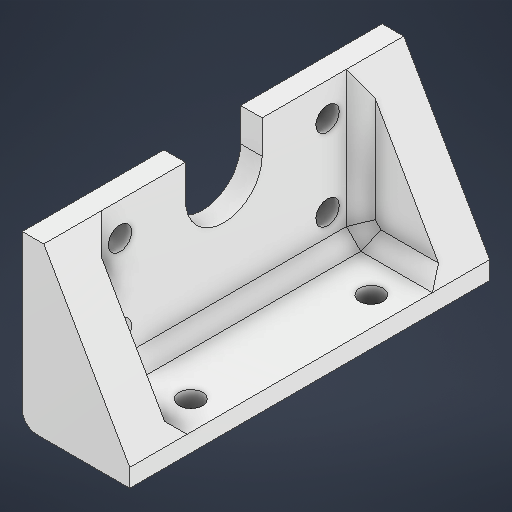
# Autodesk Inventor part: CNC-022-XAxisBallScrewStabilizerMount
Saved by Autodesk Inventor 2026.2 (Build 302298000, 298)
## iProperties
Created: 2026-06-24
Part Number: CNC-022-XAxisBallScrewStabilizerMount
Material: ABS Plastic
Document SubType Name: Modeling
Designer: Kenji
Density: 1.06 g/cm^3
Appearance: Smooth - White
Author: Kenji
Autodesk Inventor part; units mm, degrees
ref_plane "YZ Plane" through (0, 0, 0) normal (1, 0, 0) x (0, 1, 0)
ref_plane "XZ Plane" through (0, 0, 0) normal (0, 1, 0) x (-1, 0, 0)
ref_plane "XY Plane" through (0, 0, 0) normal (0, 0, 1) x (1, 0, 0)
sketch "Sketch1" plane through (0, 0, 0) normal (1, 0, 0) x (0, 1, 0)
  line L0 (-9, -23) -> (9, -23) construction
  line L1 (9, -23) -> (9, 23) construction
  line L2 (9, 23) -> (-9, 23) construction
  line L3 (-9, 23) -> (-9, -23) construction
  line L4 (-9, -23) -> (9, 23) construction
  line L5 (9, -23) -> (-9, 23) construction
  circle A0 centre (9, 23) radius 2.6
  circle A1 centre (9, -23) radius 2.6
  circle A2 centre (-9, -23) radius 2.6
  circle A3 centre (-9, 23) radius 2.6
  circle A4 centre (9, 23) radius 7.3625 construction
  circle A5 centre (9, -23) radius 7.3625 construction
  circle A6 centre (-9, -23) radius 7.3625 construction
  circle A7 centre (-9, 23) radius 7.3625 construction
  line L6 (16.3625, 30.3625) -> (-21, 30.3625)
  line L7 (-21, 30.3625) -> (-21, -30.3625)
  line L8 (-21, -30.3625) -> (16.3625, -30.3625)
  line L9 (16.3625, -30.3625) -> (16.3625, 30.3625)
  point P0 (0, 0)
  dimension "d0" = 5.2
  dimension "d1" = 46
  dimension "d2" = 18
  dimension "d3" = 4.7625
  dimension "d7" = 12
  constraints: 20 end point, 8 centre point, 7 coincident, 6 equal radius, 4 parallel, 3 tangent, 2 horizontal, 2 midpoint, 2 perpendicular
  measures "d0" diameter of A0
  measures "d1" distance of L0.end L1.end
  measures "d2" distance of L2.end L1.end
  measures "d3" radial gap between concentric circles of A4 A0
  measures "d7" distance from line of L7 L0.start
extrude "Extrusion1" add sketch "Sketch1" along normal blind 4.7625
sketch "Sketch4" plane through (4.7625, 0, 0) normal (1, 0, 0) x (0, 0, -1)
  arc A0 (-8.5, 9) -> (8.5, 9) centre (0, 9) ccw
  circle A1 centre (-23, 9) radius 2.6 projected
  line L0 (8.5, 9) -> (8.5, 16.3625)
  line L1 (30.3625, 16.3625) -> (-30.3625, 16.3625) projected
  line L2 (-8.5, 9) -> (-8.5, 16.3625)
  point P0 (0, 0)
  point P1 (27.1875, 16.3625)
  point P2 (-27.1875, 16.3625)
  dimension "d21" = 17
  constraints: 4 end point, 2 point on circle, 2 point on line, 2 tangent, 1 centre point, 1 horizontal alignment, 1 perpendicular, 1 vertical, 1 vertical alignment
  measures "d21" diameter of A0
extrude "Extrusion5" cut sketch "Sketch4" against normal through all contours L2 L1 L0 A0
sketch "Sketch5" plane through (4.7625, 0, 0) normal (1, 0, 0) x (0, 0, -1)
  line L0 (30.3625, 16.3625) -> (8.5, 16.3625) projected
  line L1 (-30.3625, 16.3625) -> (-30.3625, -21) projected
  line L2 (-30.3625, -21) -> (30.3625, -21) projected
  line L3 (30.3625, -21) -> (30.3625, 16.3625) projected
  line L4 (-8.5, 16.3625) -> (-30.3625, 16.3625) projected
  line L5 (8.5, 16.3625) -> (8.5, 9) projected
  arc A0 (-8.5, 9) -> (8.5, 9) centre (0, 9) ccw projected
  line L6 (-8.5, 9) -> (-8.5, 16.3625) projected
  circle A1 centre (-23, -9) radius 2.6 projected
  circle A2 centre (23, -9) radius 2.6 projected
  circle A3 centre (23, 9) radius 2.6 projected
  circle A4 centre (-23, 9) radius 2.6 projected
  line L7 (30.3625, -21) -> (30.3625, 13.1875) projected
  line L8 (-30.3625, -21) -> (30.3625, -21)
  line L9 (30.3625, -21) -> (30.3625, -17)
  line L10 (30.3625, -17) -> (-30.3625, -17)
  line L11 (-30.3625, -17) -> (-30.3625, -21)
  point P0 (0, 0)
  point P1 (30.3625, -17.825)
  point P2 (30.3625, -17)
  point P3 (-30.3625, -17)
  dimension "d29" = 4
  constraints: 8 end point, 2 parallel, 1 horizontal, 1 perpendicular, 1 point on line
  measures "d29" distance between parallel lines of L2 L10
extrude "Extrusion6" add sketch "Sketch5" along normal blind 19.05 contours L3 L2 L1 L10
sketch "Sketch6" plane through (4.7625, -17, 30.3625) normal (0, 1, 0) x (1, 0, 0)
  circle A0 centre (12.7, 10.3625) radius 2.6
  circle A1 centre (12.7, 50.3625) radius 2.6
  line L0 (0, 9.9625) -> (0, 4.7625) projected
  line L1 (0, 0) -> (0, 60.725) projected
  line L2 (19.05, 60.725) -> (19.05, 0) projected
  point P0 (-4.7625, 30.3625)
  point P1 (19.05, 30.3625)
  point P2 (19.05, 30.3625)
  dimension "d32" = 5.2
  dimension "d34" = 20
  dimension "d35" = 20
  dimension "d40" = 6.35
  constraints: 2 centre point, 2 midpoint, 1 equal radius, 1 vertical alignment
  measures "d32" diameter of A0
  measures "d34" vertical distance of point (19.05, 30.362) A1.centre
  measures "d35" vertical distance of point (19.05, 30.362) A0.centre
  measures "d40" distance from line of L2 A1.centre
extrude "Extrusion7" cut sketch "Sketch6" against normal through all
sketch "Sketch12" plane through (0, -21, -30.3625) normal (0, 0, -1) x (-1, 0, 0)
  line L0 (0, 0) -> (0, 37.3625) projected
  line L1 (0, 37.3625) -> (-4.7625, 37.3625) projected
  line L2 (-4.7625, 4) -> (-4.7625, 37.3625) projected
  line L3 (-4.7625, 4) -> (-23.8125, 4) projected
  line L4 (-23.8125, 0) -> (-23.8125, 4) projected
  line L5 (0, 0) -> (-23.8125, 0) projected
  line L6 (-23.8125, 0) -> (-23.8125, 4) projected
  line L7 (-4.7625, 37.3625) -> (-23.8125, 4)
  point P0 (0, 21)
  constraints: 2 end point
extrude "Extrusion13" add sketch "Sketch12" along normal blind 9.525
sketch "Sketch13" plane through (0, -21, 30.3625) normal (0, 0, 1) x (1, 0, 0)
  line L0 (4.7625, 4) -> (23.8125, 4) projected
  line L1 (4.7625, 37.3625) -> (23.8125, 4) projected
  line L2 (4.7625, 4) -> (4.7625, 37.3625) projected
  line L3 (0, 37.3625) -> (0, 0) projected
  line L4 (0, 0) -> (23.8125, 0) projected
  line L5 (23.8125, 4) -> (23.8125, 0) projected
  line L6 (4.7625, 4) -> (23.8125, 4) projected
  line L7 (4.7625, 37.3625) -> (4.7625, 4) projected
  line L8 (0, 37.3625) -> (4.7625, 37.3625) projected
  point P0 (0, 21)
  point P1 (23.8125, 4)
  point P2 (4.7625, 37.3625)
extrude "Extrusion14" add sketch "Sketch13" along normal blind 9.525
chamfer "Chamfer1" distance 3.175 angle 45 1 edges at (4.7625, -17, 0)
chamfer "Chamfer2" distance 3.175 angle 45 6 edges at (15.875, -17, 30.3625) (6.35, -15.4125, 30.3625) (4.7625, 1.2687, 30.3625) (4.7625, 1.2688, -30.3625) (6.35, -15.4125, -30.3625) (15.875, -17, -30.3625)
fillet "Fillet9" radius 3.175 1 edges at (0, -21, 0)
equation "\"d35\" = d34"
body "Solid1"
